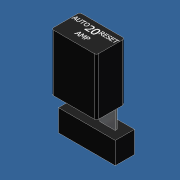
# Autodesk Inventor part: Medium CB in Holder
Saved by Autodesk Inventor 2012 (Build 160160000, 160)
## iProperties
Company: Team 801
Created: 2007-09-01
Part Number: Medium CB in Holder
Document SubType Name: Modeling
Designer: Jeffrey M
Manufacturer: Standard
Standards Organization: Custom
Mass: 4.14873 g
Surface Area: 21.3354 cm^2
Volume: 4.14873 cm^3
Density: 1 g/cm^3
Catalog Web Link: www.team801.org
Material: Default
PartAngTol0: 0.50 deg
PartAngTol1: 0.50 deg
PartAngTol2: 0.50 deg
PartLinTol0: 0.01 in
PartLinTol1: 0.01 in
PartLinTol2: 0.01 in
PartLinTol3: 0.005 in
PartAngTol3: 0deg30'
Author: Jeffrey M
Autodesk Inventor part; units mm, degrees
ref_plane "YZ Plane (RIGHT)" through (0, 0, 0) normal (1, 0, 0) x (0, 1, 0)
ref_plane "XZ Plane (TOP)" through (0, 0, 0) normal (0, 1, 0) x (-1, 0, 0)
ref_plane "XY Plane (FRONT)" through (0, 0, 0) normal (0, 0, 1) x (1, 0, 0)
sketch "Sketch2" plane through (0, 0, 0) normal (0, 1, 0) x (-1, 0, 0)
  line L0 (-12.8509, 0) -> (9.6382, 0) construction
  line L1 (0, -6.133) -> (0, 8.1773) construction
  line L2 (-7.112, 4.953) -> (7.112, 4.953)
  line L3 (7.874, 4.191) -> (7.874, -4.191)
  line L4 (7.112, -4.953) -> (-7.112, -4.953)
  line L5 (-7.874, -4.191) -> (-7.874, 4.191)
  arc A0 (-7.112, 4.953) -> (-7.874, 4.191) centre (-7.112, 4.191) ccw
  arc A1 (7.874, 4.191) -> (7.112, 4.953) centre (7.112, 4.191) ccw
  arc A2 (7.112, -4.953) -> (7.874, -4.191) centre (7.112, -4.191) ccw
  arc A3 (-7.874, -4.191) -> (-7.112, -4.953) centre (-7.112, -4.191) ccw
  point P0 (-7.874, 4.953)
  point P1 (7.874, -4.953)
  point P2 (7.874, 4.953)
  dimension "d0" = 15.748
  dimension "d1" = 9.906
  dimension "d2" = 0.762
  constraints: 8 end point, 8 point on circle, 8 tangent, 6 point on line, 4 centre point, 3 equal radius, 2 parallel, 1 horizontal, 1 perpendicular, 2 other
  measures "d0" distance of point (-7.874, 4.953) point (7.874, 4.953)
  measures "d1" distance of point (7.874, 4.953) point (7.874, -4.953)
  measures "d2" radius of A0
extrude "Extrusion1" add sketch "Sketch2" along normal blind 19.812
sketch "Sketch3" plane through (0, 0, 0) normal (0, -1, 0) x (1, 0, 0)
  line L0 (-7.112, 4.953) -> (7.112, 4.953) projected
  line L1 (-6.8707, -2.5654) -> (-1.4859, -2.5654)
  line L2 (-1.4859, -2.5654) -> (-1.4859, -3.2766)
  line L3 (-1.4859, -3.2766) -> (-6.8707, -3.2766)
  line L4 (-6.8707, -3.2766) -> (-6.8707, -2.5654)
  line L5 (1.4859, -2.5654) -> (6.8707, -2.5654)
  line L6 (6.8707, -2.5654) -> (6.8707, -3.2766)
  line L7 (6.8707, -3.2766) -> (1.4859, -3.2766)
  line L8 (1.4859, -3.2766) -> (1.4859, -2.5654)
  line L9 (0, 7.9248) -> (0, -5.9436) construction
  line L10 (1.4859, -2.921) -> (6.8707, -2.921) construction
  dimension "d5" = 0.7112
  dimension "d6" = 5.3848
  dimension "d7" = 7.874
  dimension "d8" = 2.9718
  constraints: 18 end point, 4 parallel, 2 horizontal, 2 midpoint, 2 perpendicular, 4 other
  measures "d5" distance between parallel lines of L3 L1
  measures "d6" distance of L1.start L1.end
  measures "d7" distance between parallel lines of L0 L10
  measures "d8" distance between parallel lines of L8 L2
extrude "Extrusion2" add sketch "Sketch3" along normal blind 14.478
sketch "Sketch4" plane through (0, 0, 0) normal (1, 0, 0) x (0, 1, 0)
  line L0 (-14.478, -2.5654) -> (-14.478, -3.2766) projected
  line L1 (19.812, -4.191) -> (19.812, 4.191) projected
  line L2 (-14.8844, 0.4318) -> (-7.2644, 0.4318)
  line L3 (-7.2644, 0.4318) -> (-7.2644, -6.2738)
  line L4 (-7.2644, -6.2738) -> (-14.8844, -6.2738)
  line L5 (-14.8844, -6.2738) -> (-14.8844, 0.4318)
  line L6 (-14.478, -2.921) -> (-12.4968, -2.921) construction
  point P0 (0, 0)
  dimension "d11" = 34.6964
  dimension "d12" = 6.7056
  dimension "d13" = 7.62
  constraints: 10 end point, 2 parallel, 2 perpendicular, 1 horizontal, 1 midpoint, 1 other
  measures "d11" distance between parallel lines of L1 L5
  measures "d12" distance of L4.end L2.start
  measures "d13" distance of L2.start L2.end
extrude "Extrusion3" add sketch "Sketch4" along normal mid plane 19.812
sketch "Sketch5" plane through (0, 19.812, 0) normal (0, 1, 0) x (1, 0, 0)
  line L0 (-10.1366, 3.2132) -> (9.6153, 3.2132) construction
  line L1 (9.6153, 3.2132) -> (9.6153, -3.7199) construction
  line L2 (9.6153, -3.7199) -> (-10.1366, -3.7199) construction
  line L3 (-10.1366, -3.7199) -> (-10.1366, 3.2132) construction
  line L4 (-11.2885, 3.3094) -> (11.4388, 3.3094) construction
  line L5 (11.4388, 3.3094) -> (11.4388, 1.6453) construction
  line L6 (11.4388, 1.6453) -> (-11.2885, 1.6453) construction
  line L7 (-11.2885, 1.6453) -> (-11.2885, 3.3094) construction
  line L8 (-7.5899, 1.7533) -> (-7.0762, 3.2773)
  line L9 (-7.0762, 3.2773) -> (-6.8267, 3.2773)
  line L10 (-6.8267, 3.2773) -> (-6.3129, 1.7533)
  line L11 (-6.3129, 1.7533) -> (-6.5266, 1.7533)
  line L12 (-6.5266, 1.7533) -> (-6.6649, 2.1794)
  line L13 (-6.6649, 2.1794) -> (-7.2466, 2.1794)
  line L14 (-7.2466, 2.1794) -> (-7.3849, 1.7533)
  line L15 (-7.3849, 1.7533) -> (-7.5899, 1.7533)
  line L16 (-6.7205, 2.3523) -> (-6.9564, 3.0698)
  line L17 (-6.9564, 3.0698) -> (-7.191, 2.3523)
  line L18 (-7.191, 2.3523) -> (-6.7205, 2.3523)
  spline S0 degree 2 poles (-5.6361, 1.7212) (-5.7708, 1.7212) (-5.9708, 1.7916) (-6.0412, 1.862) knots 0 0 0 1 2 2 2
  spline S1 degree 2 poles (-6.0412, 1.862) (-6.1215, 1.941) (-6.187, 2.1633) (-6.187, 2.3264) knots 0 0 0 1 2 2 2
  line L19 (-6.187, 2.3264) -> (-6.187, 3.2773)
  line L20 (-6.187, 3.2773) -> (-5.9844, 3.2773)
  line L21 (-5.9844, 3.2773) -> (-5.9844, 2.3264)
  spline S2 degree 2 poles (-5.9844, 2.3264) (-5.9844, 2.2202) (-5.9572, 2.0769) (-5.919, 2.0188) knots 0 0 0 1 2 2 2
  spline S3 degree 2 poles (-5.919, 2.0188) (-5.8782, 1.9571) (-5.7374, 1.8941) (-5.6361, 1.8941) knots 0 0 0 1 2 2 2
  spline S4 degree 2 poles (-5.6361, 1.8941) (-5.541, 1.8941) (-5.3928, 1.9571) (-5.3521, 2.0188) knots 0 0 0 1 2 2 2
  spline S5 degree 2 poles (-5.3521, 2.0188) (-5.3138, 2.0769) (-5.2866, 2.2189) (-5.2866, 2.3214) knots 0 0 0 1 2 2 2
  line L22 (-5.2866, 2.3214) -> (-5.2866, 3.2773)
  line L23 (-5.2866, 3.2773) -> (-5.0841, 3.2773)
  line L24 (-5.0841, 3.2773) -> (-5.0841, 2.3264)
  spline S6 degree 2 poles (-5.0841, 2.3264) (-5.0841, 2.167) (-5.1483, 1.9398) (-5.2298, 1.862) knots 0 0 0 1 2 2 2
  spline S7 degree 2 poles (-5.2298, 1.862) (-5.3027, 1.7904) (-5.4953, 1.7212) (-5.6361, 1.7212) knots 0 0 0 1 2 2 2
  line L25 (-4.4382, 1.7533) -> (-4.4382, 3.097)
  line L26 (-4.4382, 3.097) -> (-4.9495, 3.097)
  line L27 (-4.9495, 3.097) -> (-4.9495, 3.2773)
  line L28 (-4.9495, 3.2773) -> (-3.7243, 3.2773)
  line L29 (-3.7243, 3.2773) -> (-3.7243, 3.097)
  line L30 (-3.7243, 3.097) -> (-4.2356, 3.097)
  line L31 (-4.2356, 3.097) -> (-4.2356, 1.7533)
  line L32 (-4.2356, 1.7533) -> (-4.4382, 1.7533)
  spline S8 degree 2 poles (-2.4918, 3.1032) (-2.4054, 3.0019) (-2.309, 2.7055) (-2.309, 2.5153) knots 0 0 0 1 2 2 2
  spline S9 degree 2 poles (-2.309, 2.5153) (-2.309, 2.3301) (-2.4029, 2.03) (-2.4918, 1.9287) knots 0 0 0 1 2 2 2
  spline S10 degree 2 poles (-2.4918, 1.9287) (-2.5857, 1.8225) (-2.8339, 1.7212) (-2.9833, 1.7212) knots 0 0 0 1 2 2 2
  spline S11 degree 2 poles (-2.9833, 1.7212) (-3.1377, 1.7212) (-3.3847, 1.8262) (-3.4749, 1.9287) knots 0 0 0 1 2 2 2
  spline S12 degree 2 poles (-3.4749, 1.9287) (-3.5626, 2.03) (-3.6564, 2.3276) (-3.6564, 2.5153) knots 0 0 0 1 2 2 2
  spline S13 degree 2 poles (-3.6564, 2.5153) (-3.6564, 2.7067) (-3.5613, 2.9982) (-3.4736, 3.1032) knots 0 0 0 1 2 2 2
  spline S14 degree 2 poles (-3.4736, 3.1032) (-3.3847, 3.2045) (-3.1365, 3.3094) (-2.9833, 3.3094) knots 0 0 0 1 2 2 2
  spline S15 degree 2 poles (-2.9833, 3.3094) (-2.8277, 3.3094) (-2.5783, 3.2007) (-2.4918, 3.1032) knots 0 0 0 1 2 2 2
  spline S16 degree 2 poles (-2.5202, 2.5153) (-2.5202, 2.666) (-2.5857, 2.8994) (-2.6449, 2.976) knots 0 0 0 1 2 2 2
  spline S17 degree 2 poles (-2.6449, 2.976) (-2.7055, 3.055) (-2.8759, 3.1341) (-2.9821, 3.1341) knots 0 0 0 1 2 2 2
  spline S18 degree 2 poles (-2.9821, 3.1341) (-3.092, 3.1341) (-3.2575, 3.0575) (-3.3205, 2.976) knots 0 0 0 1 2 2 2
  spline S19 degree 2 poles (-3.3205, 2.976) (-3.381, 2.8982) (-3.4452, 2.6635) (-3.4452, 2.5153) knots 0 0 0 1 2 2 2
  spline S20 degree 2 poles (-3.4452, 2.5153) (-3.4452, 2.2152) (-3.1933, 1.8966) (-2.9821, 1.8966) knots 0 0 0 1 2 2 2
  spline S21 degree 2 poles (-2.9821, 1.8966) (-2.7709, 1.8966) (-2.5202, 2.2152) (-2.5202, 2.5153) knots 0 0 0 1 2 2 2
  line L33 (3.02, 1.7533) -> (2.757, 1.7533)
  line L34 (2.757, 1.7533) -> (2.2753, 2.3597)
  line L35 (2.2753, 2.3597) -> (2.0431, 2.3597)
  line L36 (2.0431, 2.3597) -> (2.0431, 1.7533)
  line L37 (2.0431, 1.7533) -> (1.8406, 1.7533)
  line L38 (1.8406, 1.7533) -> (1.8406, 3.2773)
  line L39 (1.8406, 3.2773) -> (2.2333, 3.2773)
  spline S22 degree 2 poles (2.2333, 3.2773) (2.3642, 3.2773) (2.5409, 3.2489) (2.6211, 3.197) knots 0 0 0 1 2 2 2
  spline S23 degree 2 poles (2.6211, 3.197) (2.7014, 3.1452) (2.794, 2.9834) (2.794, 2.8636) knots 0 0 0 1 2 2 2
  spline S24 degree 2 poles (2.794, 2.8636) (2.794, 2.6969) (2.6236, 2.4709) (2.4779, 2.4165) knots 0 0 0 1 2 2 2
  line L40 (2.4779, 2.4165) -> (3.02, 1.7533)
  spline S25 degree 2 poles (2.5828, 2.8475) (2.5828, 2.9142) (2.5359, 3.0167) (2.4865, 3.0501) knots 0 0 0 1 2 2 2
  spline S26 degree 2 poles (2.4865, 3.0501) (2.4433, 3.0785) (2.3284, 3.1019) (2.2445, 3.1019) knots 0 0 0 1 2 2 2
  line L41 (2.2445, 3.1019) -> (2.0431, 3.1019)
  line L42 (2.0431, 3.1019) -> (2.0431, 2.5289)
  line L43 (2.0431, 2.5289) -> (2.221, 2.5289)
  spline S27 degree 2 poles (2.221, 2.5289) (2.3087, 2.5289) (2.4482, 2.5598) (2.4964, 2.6079) knots 0 0 0 1 2 2 2
  spline S28 degree 2 poles (2.4964, 2.6079) (2.5409, 2.6499) (2.5828, 2.7685) (2.5828, 2.8475) knots 0 0 0 1 2 2 2
  line L44 (3.1411, 1.7533) -> (3.1411, 3.2773)
  line L45 (3.1411, 3.2773) -> (4.0945, 3.2773)
  line L46 (4.0945, 3.2773) -> (4.0945, 3.097)
  line L47 (4.0945, 3.097) -> (3.3436, 3.097)
  line L48 (3.3436, 3.097) -> (3.3436, 2.6796)
  line L49 (3.3436, 2.6796) -> (4.0439, 2.6796)
  line L50 (4.0439, 2.6796) -> (4.0439, 2.4993)
  line L51 (4.0439, 2.4993) -> (3.3436, 2.4993)
  line L52 (3.3436, 2.4993) -> (3.3436, 1.9336)
  line L53 (3.3436, 1.9336) -> (4.0945, 1.9336)
  line L54 (4.0945, 1.9336) -> (4.0945, 1.7533)
  line L55 (4.0945, 1.7533) -> (3.1411, 1.7533)
  spline S29 degree 2 poles (4.7416, 1.7261) (4.5761, 1.7261) (4.344, 1.7953) (4.2415, 1.8447) knots 0 0 0 1 2 2 2
  line L56 (4.2415, 1.8447) -> (4.2415, 2.0991)
  line L57 (4.2415, 2.0991) -> (4.2563, 2.0991)
  spline S30 degree 2 poles (4.2563, 2.0991) (4.3563, 2.0053) (4.6095, 1.9015) (4.7268, 1.9015) knots 0 0 0 1 2 2 2
  spline S31 degree 2 poles (4.7268, 1.9015) (4.8948, 1.9015) (5.0664, 2.0411) (5.0664, 2.1559) knots 0 0 0 1 2 2 2
  spline S32 degree 2 poles (5.0664, 2.1559) (5.0664, 2.2473) (4.9763, 2.3609) (4.8787, 2.3893) knots 0 0 0 1 2 2 2
  spline S33 degree 2 poles (4.8787, 2.3893) (4.8083, 2.4091) (4.691, 2.4363) (4.6033, 2.4585) knots 0 0 0 1 2 2 2
  spline S34 degree 2 poles (4.6033, 2.4585) (4.5243, 2.4795) (4.3995, 2.5425) (4.3514, 2.5931) knots 0 0 0 1 2 2 2
  spline S35 degree 2 poles (4.3514, 2.5931) (4.3044, 2.6438) (4.2526, 2.7796) (4.2526, 2.8685) knots 0 0 0 1 2 2 2
  spline S36 degree 2 poles (4.2526, 2.8685) (4.2526, 3.0538) (4.5416, 3.3045) (4.7651, 3.3045) knots 0 0 0 1 2 2 2
  spline S37 degree 2 poles (4.7651, 3.3045) (4.8935, 3.3045) (5.1208, 3.2539) (5.2183, 3.2057) knots 0 0 0 1 2 2 2
  line L58 (5.2183, 3.2057) -> (5.2183, 2.9636)
  line L59 (5.2183, 2.9636) -> (5.2035, 2.9636)
  spline S38 degree 2 poles (5.2035, 2.9636) (5.1307, 3.0303) (4.9034, 3.1291) (4.7787, 3.1291) knots 0 0 0 1 2 2 2
  spline S39 degree 2 poles (4.7787, 3.1291) (4.6379, 3.1291) (4.4638, 2.997) (4.4638, 2.8895) knots 0 0 0 1 2 2 2
  spline S40 degree 2 poles (4.4638, 2.8895) (4.4638, 2.7932) (4.5663, 2.6783) (4.6626, 2.6524) knots 0 0 0 1 2 2 2
  spline S41 degree 2 poles (4.6626, 2.6524) (4.7268, 2.6351) (4.9133, 2.5907) (4.9751, 2.5721) knots 0 0 0 1 2 2 2
  spline S42 degree 2 poles (4.9751, 2.5721) (5.1319, 2.524) (5.2776, 2.3301) (5.2776, 2.188) knots 0 0 0 1 2 2 2
  spline S43 degree 2 poles (5.2776, 2.188) (5.2776, 2.0979) (5.2048, 1.925) (5.1393, 1.8645) knots 0 0 0 1 2 2 2
  spline S44 degree 2 poles (5.1393, 1.8645) (5.0664, 1.7978) (4.8812, 1.7261) (4.7416, 1.7261) knots 0 0 0 1 2 2 2
  line L60 (5.4839, 1.7533) -> (5.4839, 3.2773)
  line L61 (5.4839, 3.2773) -> (6.4373, 3.2773)
  line L62 (6.4373, 3.2773) -> (6.4373, 3.097)
  line L63 (6.4373, 3.097) -> (5.6864, 3.097)
  line L64 (5.6864, 3.097) -> (5.6864, 2.6796)
  line L65 (5.6864, 2.6796) -> (6.3867, 2.6796)
  line L66 (6.3867, 2.6796) -> (6.3867, 2.4993)
  line L67 (6.3867, 2.4993) -> (5.6864, 2.4993)
  line L68 (5.6864, 2.4993) -> (5.6864, 1.9336)
  line L69 (5.6864, 1.9336) -> (6.4373, 1.9336)
  line L70 (6.4373, 1.9336) -> (6.4373, 1.7533)
  line L71 (6.4373, 1.7533) -> (5.4839, 1.7533)
  line L72 (7.0153, 1.7533) -> (7.0153, 3.097)
  line L73 (7.0153, 3.097) -> (6.504, 3.097)
  line L74 (6.504, 3.097) -> (6.504, 3.2773)
  line L75 (6.504, 3.2773) -> (7.7291, 3.2773)
  line L76 (7.7291, 3.2773) -> (7.7291, 3.097)
  line L77 (7.7291, 3.097) -> (7.2178, 3.097)
  line L78 (7.2178, 3.097) -> (7.2178, 1.7533)
  line L79 (7.2178, 1.7533) -> (7.0153, 1.7533)
  line L80 (-0.415, 0.6197) -> (-1.9814, 0.6197)
  line L81 (-1.9814, 0.6197) -> (-1.9814, 0.9799)
  spline S45 degree 2 poles (-1.9814, 0.9799) (-1.8126, 1.1384) (-1.5121, 1.4327) (-1.368, 1.5912) knots 0 0 0 1 2 2 2
  spline S46 degree 2 poles (-1.368, 1.5912) (-1.0778, 1.9102) (-0.8658, 2.2931) (-0.8658, 2.4969) knots 0 0 0 1 2 2 2
  spline S47 degree 2 poles (-0.8658, 2.4969) (-0.8658, 2.6039) (-0.9316, 2.7645) (-0.9913, 2.8159) knots 0 0 0 1 2 2 2
  spline S48 degree 2 poles (-0.9913, 2.8159) (-1.051, 2.8674) (-1.2074, 2.9188) (-1.3021, 2.9188) knots 0 0 0 1 2 2 2
  spline S49 degree 2 poles (-1.3021, 2.9188) (-1.3927, 2.9188) (-1.578, 2.8736) (-1.6623, 2.8386) knots 0 0 0 1 2 2 2
  spline S50 degree 2 poles (-1.6623, 2.8386) (-1.7344, 2.8097) (-1.8682, 2.7274) (-1.9093, 2.6986) knots 0 0 0 1 2 2 2
  line L82 (-1.9093, 2.6986) -> (-1.9279, 2.6986)
  line L83 (-1.9279, 2.6986) -> (-1.9279, 3.0609)
  spline S51 degree 2 poles (-1.9279, 3.0609) (-1.8229, 3.1123) (-1.4462, 3.2132) (-1.2774, 3.2132) knots 0 0 0 1 2 2 2
  spline S52 degree 2 poles (-1.2774, 3.2132) (-0.9213, 3.2132) (-0.52, 2.8365) (-0.52, 2.5154) knots 0 0 0 1 2 2 2
  spline S53 degree 2 poles (-0.52, 2.5154) (-0.52, 2.3651) (-0.5899, 2.114) (-0.6517, 2.007) knots 0 0 0 1 2 2 2
  spline S54 degree 2 poles (-0.6517, 2.007) (-0.7134, 1.8958) (-0.8925, 1.6777) (-0.9913, 1.5727) knots 0 0 0 1 2 2 2
  spline S55 degree 2 poles (-0.9913, 1.5727) (-1.1519, 1.3977) (-1.545, 1.0231) (-1.6623, 0.914) knots 0 0 0 1 2 2 2
  line L84 (-1.6623, 0.914) -> (-0.415, 0.914)
  line L85 (-0.415, 0.914) -> (-0.415, 0.6197)
  spline S56 degree 2 poles (1.5055, 1.8897) (1.5055, 1.2063) (1.1082, 0.5661) (0.6945, 0.5661) knots 0 0 0 1 2 2 2
  spline S57 degree 2 poles (0.6945, 0.5661) (0.2746, 0.5661) (-0.1186, 1.2186) (-0.1186, 1.8876) knots 0 0 0 1 2 2 2
  spline S58 degree 2 poles (-0.1186, 1.8876) (-0.1186, 2.5751) (0.2787, 3.2111) (0.6945, 3.2111) knots 0 0 0 1 2 2 2
  spline S59 degree 2 poles (0.6945, 3.2111) (1.1123, 3.2111) (1.5055, 2.5525) (1.5055, 1.8897) knots 0 0 0 1 2 2 2
  spline S60 degree 2 poles (1.0691, 1.1157) (1.1185, 1.2413) (1.1596, 1.6283) (1.1596, 1.8897) knots 0 0 0 1 2 2 2
  spline S61 degree 2 poles (1.1596, 1.8897) (1.1596, 2.1511) (1.1185, 2.536) (1.067, 2.6657) knots 0 0 0 1 2 2 2
  spline S62 degree 2 poles (1.067, 2.6657) (1.0156, 2.7953) (0.8365, 2.9291) (0.6945, 2.9291) knots 0 0 0 1 2 2 2
  spline S63 degree 2 poles (0.6945, 2.9291) (0.5524, 2.9291) (0.3692, 2.7953) (0.3157, 2.6615) knots 0 0 0 1 2 2 2
  spline S64 degree 2 poles (0.3157, 2.6615) (0.2643, 2.5319) (0.2272, 2.1367) (0.2272, 1.8876) knots 0 0 0 1 2 2 2
  spline S65 degree 2 poles (0.2272, 1.8876) (0.2272, 1.62) (0.2602, 1.2619) (0.3137, 1.1219) knots 0 0 0 1 2 2 2
  spline S66 degree 2 poles (0.3137, 1.1219) (0.3631, 0.9902) (0.5463, 0.8481) (0.6945, 0.8481) knots 0 0 0 1 2 2 2
  spline S67 degree 2 poles (0.6945, 0.8481) (0.8344, 0.8481) (1.0176, 0.9819) (1.0691, 1.1157) knots 0 0 0 1 2 2 2
  line L86 (-2.4535, -2.4417) -> (-1.8969, -0.7907)
  line L87 (-1.8969, -0.7907) -> (-1.6266, -0.7907)
  line L88 (-1.6266, -0.7907) -> (-1.0701, -2.4417)
  line L89 (-1.0701, -2.4417) -> (-1.3015, -2.4417)
  line L90 (-1.3015, -2.4417) -> (-1.4514, -1.9801)
  line L91 (-1.4514, -1.9801) -> (-2.0815, -1.9801)
  line L92 (-2.0815, -1.9801) -> (-2.2314, -2.4417)
  line L93 (-2.2314, -2.4417) -> (-2.4535, -2.4417)
  line L94 (-1.5116, -1.7928) -> (-1.7671, -1.0155)
  line L95 (-1.7671, -1.0155) -> (-2.0213, -1.7928)
  line L96 (-2.0213, -1.7928) -> (-1.5116, -1.7928)
  line L97 (0.502, -2.4417) -> (0.2826, -2.4417)
  line L98 (0.2826, -2.4417) -> (0.2826, -1.0195)
  line L99 (0.2826, -1.0195) -> (-0.1482, -1.9868)
  line L100 (-0.1482, -1.9868) -> (-0.282, -1.9868)
  line L101 (-0.282, -1.9868) -> (-0.7088, -1.0195)
  line L102 (-0.7088, -1.0195) -> (-0.7088, -2.4417)
  line L103 (-0.7088, -2.4417) -> (-0.9135, -2.4417)
  line L104 (-0.9135, -2.4417) -> (-0.9135, -0.7907)
  line L105 (-0.9135, -0.7907) -> (-0.6138, -0.7907)
  line L106 (-0.6138, -0.7907) -> (-0.2017, -1.7099)
  line L107 (-0.2017, -1.7099) -> (0.197, -0.7907)
  line L108 (0.197, -0.7907) -> (0.502, -0.7907)
  line L109 (0.502, -0.7907) -> (0.502, -2.4417)
  spline S68 degree 2 poles (1.8801, -1.2884) (1.8801, -1.3955) (1.8038, -1.5881) (1.7356, -1.655) knots 0 0 0 1 2 2 2
  spline S69 degree 2 poles (1.7356, -1.655) (1.6499, -1.7393) (1.4185, -1.8263) (1.2419, -1.8263) knots 0 0 0 1 2 2 2
  line L110 (1.2419, -1.8263) -> (1.0559, -1.8263)
  line L111 (1.0559, -1.8263) -> (1.0559, -2.4417)
  line L112 (1.0559, -2.4417) -> (0.8365, -2.4417)
  line L113 (0.8365, -2.4417) -> (0.8365, -0.7907)
  line L114 (0.8365, -0.7907) -> (1.2512, -0.7907)
  spline S70 degree 2 poles (1.2512, -0.7907) (1.3984, -0.7907) (1.6045, -0.8389) (1.6834, -0.8937) knots 0 0 0 1 2 2 2
  spline S71 degree 2 poles (1.6834, -0.8937) (1.7757, -0.9566) (1.8801, -1.1506) (1.8801, -1.2884) knots 0 0 0 1 2 2 2
  spline S72 degree 2 poles (1.6513, -1.2951) (1.6513, -1.2095) (1.5924, -1.0837) (1.5322, -1.0436) knots 0 0 0 1 2 2 2
  spline S73 degree 2 poles (1.5322, -1.0436) (1.48, -1.0088) (1.3409, -0.9807) (1.2379, -0.9807) knots 0 0 0 1 2 2 2
  line L115 (1.2379, -0.9807) -> (1.0559, -0.9807)
  line L116 (1.0559, -0.9807) -> (1.0559, -1.639)
  line L117 (1.0559, -1.639) -> (1.2058, -1.639)
  spline S74 degree 2 poles (1.2058, -1.639) (1.3395, -1.639) (1.5041, -1.5962) (1.5576, -1.54) knots 0 0 0 1 2 2 2
  spline S75 degree 2 poles (1.5576, -1.54) (1.6071, -1.4905) (1.6513, -1.3741) (1.6513, -1.2951) knots 0 0 0 1 2 2 2
  constraints: 4 other
extrude "Extrusion4" cut sketch "Sketch5" against normal blind 0.0025
body "Solid1"
